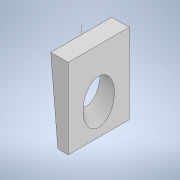
# Autodesk Inventor part: waterHeaterVent-V02
Saved by Autodesk Inventor 2021.1 (Build 251245010, 245A)
## iProperties
Created: 2020-10-25
Part Number: waterHeaterVent-V02
Material: Generic
Document SubType Name: Modeling
Designer: robst
Density: 1 g/cm^3
Appearance: Default
Author: robst
Autodesk Inventor part; units mm, degrees
ref_plane "YZ Plane" through (0, 0, 0) normal (1, 0, 0) x (0, 1, 0)
ref_plane "XZ Plane" through (0, 0, 0) normal (0, 1, 0) x (-1, 0, 0)
ref_plane "XY Plane" through (0, 0, 0) normal (0, 0, 1) x (1, 0, 0)
sketch "Sketch1" plane through (0, 0, 0) normal (0, 0, 1) x (1, 0, 0)
  line L0 (0, 0) -> (5.1111, -58.42)
  line L1 (0, -70.104) -> (0, 11.684) projected
  line L2 (0, 0) -> (12.7, 0)
  line L3 (12.7, 0) -> (12.7, -58.42)
  line L4 (5.1111, -58.42) -> (12.7, -58.42)
  dimension "d0" = 5
  dimension "d1" = 12.7
  dimension "d3" = 58.42
  constraints: 8 end point, 2 horizontal, 1 vertical
  measures "d0" angle of L0 L1
  measures "d1" distance of L0.start L2.end
  measures "d3" distance of L2.end L3.end
extrude "Extrusion1" add sketch "Sketch1" along normal mid plane 44.45
ref_plane "Work Plane1" through (12.7, -58.42, 0) normal (0.7071068, -0.7071068, 0) x (0, 0, 1)
sketch "Sketch2" plane through (12.7, -58.42, 0) normal (0.7071068, -0.7071068, 0) x (0, 0, 1)
  line L0 (22.225, 0) -> (22.225, -41.3092) projected
  line L1 (22.225, -41.3092) -> (-22.225, -41.3092) projected
  line L2 (-22.225, -41.3092) -> (-22.225, 0) projected
  line L3 (-22.225, 0) -> (22.225, 0) projected
  circle A0 centre (0, -15.9092) radius 11.43
  point P0 (0, -32.3289)
  dimension "d7" = 22.86
  dimension "d10" = 25.4
  constraints: 1 centre point
  measures "d7" diameter of A0
  measures "d10" distance from line of A0.centre L1
extrude "Extrusion2" cut sketch "Sketch2" against normal through all contours A0
sketch "Sketch3" plane through (5.1111, -58.42, -22.225) normal (-0.9961947, -0.0871557, 0) x (0, 0, 1)
  line L0 (0, 0) -> (0, 58.6432) construction
  line L1 (0, 8.89) -> (44.45, 8.89) construction
  line L2 (44.45, 58.6432) -> (44.45, 0) construction
  line L3 (0, 0) -> (44.45, 0) construction
  line L4 (16.6636, 13.716) -> (13.3831, 4.191)
  line L5 (13.3831, 4.191) -> (12.0169, 4.191)
  line L6 (12.0169, 4.191) -> (8.7364, 13.716)
  line L7 (8.7364, 13.716) -> (10.0949, 13.716)
  line L8 (10.0949, 13.716) -> (12.7347, 5.8042)
  line L9 (12.7347, 5.8042) -> (15.3746, 13.716)
  line L10 (15.3746, 13.716) -> (16.6636, 13.716)
  line L11 (20.9012, 7.7802) -> (17.2965, 7.7802)
  line L12 (17.2965, 7.7802) -> (17.2965, 8.9381)
  line L13 (17.2965, 8.9381) -> (20.9012, 8.9381)
  line L14 (20.9012, 8.9381) -> (20.9012, 7.7802)
  spline S0 degree 2 poles (28.0951, 8.9535) (28.0951, 6.3909) (26.6054, 3.9903) (25.0539, 3.9903) knots 0 0 0 1 2 2 2
  spline S1 degree 2 poles (25.0539, 3.9903) (23.4793, 3.9903) (22.005, 6.4372) (22.005, 8.9458) knots 0 0 0 1 2 2 2
  spline S2 degree 2 poles (22.005, 8.9458) (22.005, 11.5239) (23.4947, 13.909) (25.0539, 13.909) knots 0 0 0 1 2 2 2
  spline S3 degree 2 poles (25.0539, 13.909) (26.6209, 13.909) (28.0951, 11.439) (28.0951, 8.9535) knots 0 0 0 1 2 2 2
  spline S4 degree 2 poles (26.4588, 6.0512) (26.644, 6.5221) (26.7984, 7.9732) (26.7984, 8.9535) knots 0 0 0 1 2 2 2
  spline S5 degree 2 poles (26.7984, 8.9535) (26.7984, 9.9338) (26.644, 11.3772) (26.451, 11.8635) knots 0 0 0 1 2 2 2
  spline S6 degree 2 poles (26.451, 11.8635) (26.2581, 12.3498) (25.5865, 12.8515) (25.0539, 12.8515) knots 0 0 0 1 2 2 2
  spline S7 degree 2 poles (25.0539, 12.8515) (24.5213, 12.8515) (23.8344, 12.3498) (23.6337, 11.8481) knots 0 0 0 1 2 2 2
  spline S8 degree 2 poles (23.6337, 11.8481) (23.4407, 11.3618) (23.3018, 9.8798) (23.3018, 8.9458) knots 0 0 0 1 2 2 2
  spline S9 degree 2 poles (23.3018, 8.9458) (23.3018, 7.9423) (23.4253, 6.5993) (23.626, 6.0744) knots 0 0 0 1 2 2 2
  spline S10 degree 2 poles (23.626, 6.0744) (23.8112, 5.5804) (24.4982, 5.0478) (25.0539, 5.0478) knots 0 0 0 1 2 2 2
  spline S11 degree 2 poles (25.0539, 5.0478) (25.5788, 5.0478) (26.2658, 5.5495) (26.4588, 6.0512) knots 0 0 0 1 2 2 2
  line L15 (34.7102, 4.191) -> (30.0634, 4.191)
  line L16 (30.0634, 4.191) -> (30.0634, 5.1636)
  line L17 (30.0634, 5.1636) -> (31.7925, 5.1636)
  line L18 (31.7925, 5.1636) -> (31.7925, 11.547)
  line L19 (31.7925, 11.547) -> (30.0634, 11.547)
  line L20 (30.0634, 11.547) -> (30.0634, 12.4192)
  spline S12 degree 2 poles (30.0634, 12.4192) (31.0437, 12.4192) (31.97, 12.975) (32.0317, 13.7469) knots 0 0 0 1 2 2 2
  line L21 (32.0317, 13.7469) -> (33.0197, 13.7469)
  line L22 (33.0197, 13.7469) -> (33.0197, 5.1636)
  line L23 (33.0197, 5.1636) -> (34.7102, 5.1636)
  line L24 (34.7102, 5.1636) -> (34.7102, 4.191)
  point P0 (22.225, 58.6432)
  dimension "d12" = 8.89
  constraints: 2 end point, 2 horizontal, 2 point on line
  measures "d12" distance between parallel lines of L3 L1
extrude "Extrusion3" cut sketch "Sketch3" against normal blind 1.27
equation "\"d0\" = backAngle"
equation "\"d1\" = topPartDepth"
equation "\"d3\" = partHeight"
equation "\"d4\" = partWidth"
equation "\"d7\" = pipeExteriorDiameter"
equation "\"d10\" = pipeCenter"
equation "\"d13\" = textDepth"
equation "\"topPartDepth\" = 12.7"
equation "\"backAngle\" = 5deg"
equation "\"partHeight\" = 58.42"
equation "\"partWidth\" = 44.45"
equation "\"pipeExteriorDiameter\" = 22.86"
equation "\"pipeCenter\" = 25.4"
equation "\"filletEdge\" = 1.05833"
equation "\"textDepth\" = 1.27"
body "Solid1"
